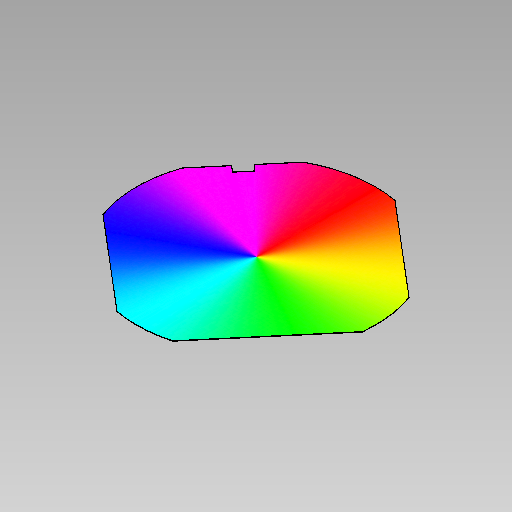
# Autodesk Inventor part: Color_wheel
Saved by Autodesk Inventor 2020 (Build 240168000, 168)
## iProperties
Created: 2019-06-06
Part Number: Color_wheel
Material: Generic
Document SubType Name: Modeling
Designer: Varga Daniel
Density: 1 g/cm^3
Appearance: Default
Author: Varga Daniel
Autodesk Inventor part; units mm, degrees
ref_plane "YZ Plane" through (0, 0, 0) normal (1, 0, 0) x (0, 1, 0)
ref_plane "XZ Plane" through (0, 0, 0) normal (0, 1, 0) x (-1, 0, 0)
ref_plane "XY Plane" through (0, 0, 0) normal (0, 0, 1) x (1, 0, 0)
sketch "Sketch1" plane through (0, 0, 0) normal (0, 1, 0) x (-1, 0, 0)
  circle A0 centre (0, 0) radius 30
  dimension "d2" = 60
  constraints: 1 centre point, 1 coincident
  measures "d2" diameter of A0
extrude "Extrusion1" add sketch "Sketch1" along normal blind 0.1
sketch "Sketch2" plane through (0, 0.1, 0) normal (0, 1, 0) x (1, 0, 0)
  circle A0 centre (0, 0) radius 30 projected
  line L0 (-44.4053, 35) -> (44.4053, 35) construction
  line L1 (44.4053, 35) -> (44.4053, -35) construction
  line L2 (44.4053, -35) -> (-44.4053, -35) construction
  line L3 (-44.4053, -35) -> (-44.4053, 35) construction
  line L4 (0, 0) -> (51.8598, 0) construction
  line L5 (0, 0) -> (0, -54.6887) construction
  dimension "d24" = 70
  constraints: 4 end point, 1 horizontal, 1 parallel, 1 perpendicular, 4 other
  measures "d24" distance between parallel lines of L2 L0
decal "Decal1"
sketch "Sketch3" plane through (0, 0.1, 0) normal (0, 1, 0) x (1, 0, 0)
  line L0 (-18.5655, 18.3118) -> (-21.1477, 15.257)
  line L1 (-18.5655, 18.3118) -> (-20.0929, 19.6029)
  line L2 (-20.0929, 19.6029) -> (-4.5996, 37.9321)
  line L3 (-4.5996, 37.9321) -> (35.7245, 3.8469)
  line L4 (35.7245, 3.8469) -> (2.1557, -35.8663)
  line L5 (2.1557, -35.8663) -> (-38.1684, -1.7811)
  line L6 (-38.1684, -1.7811) -> (-22.6751, 16.5481)
  line L7 (-21.1477, 15.257) -> (-22.6751, 16.5481)
  line L8 (-4.5996, 37.9321) -> (35.7245, 3.8469)
  line L9 (35.7245, 3.8469) -> (2.1557, -35.8663)
  line L10 (2.1557, -35.8663) -> (-38.1684, -1.7811)
  line L11 (-38.1684, -1.7811) -> (-4.5996, 37.9321)
  point P0 (0, 0)
  constraints: 24 end point, 2 parallel, 2 perpendicular, 1 collinear
extrude "Extrusion2" cut sketch "Sketch3" against normal blind 0.1 contours L1 L2 L3 L4 L5 L6 L7 L0 keep common part
body "Solid1"
